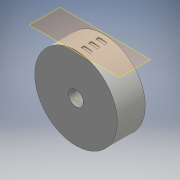
# Autodesk Inventor part: Part4
Saved by Autodesk Inventor 2016 (Build 200138000, 138)
## iProperties
Created: 2016-09-09
Part Number: Part4
Material: Generic
Document SubType Name: Modeling
Designer: Muhammad
Density: 1 g/cm^3
Appearance: Default
Author: Muhammad
Autodesk Inventor part; units mm, degrees
ref_plane "YZ Plane" through (0, 0, 0) normal (1, 0, 0) x (0, 1, 0)
ref_plane "XZ Plane" through (0, 0, 0) normal (0, 1, 0) x (-1, 0, 0)
sketch "Sketch1" plane through (0, 0, 0) normal (0, 1, 0) x (-1, 0, 0)
  circle A0 centre (0, 0) radius 14
  circle A1 centre (0, 0) radius 2.5
  dimension "d0" = 28
  dimension "d1" = 5
  constraints: 2 centre point, 2 coincident
  measures "d0" diameter of A0
  measures "d1" diameter of A1
extrude "Extrusion1" add sketch "Sketch1" along normal blind 9.5
sketch "Sketch2" plane through (0, 0, 0) normal (0, 0, 1) x (1, 0, 0)
  point P0 (0, 0)
ref_plane "Work Plane1" through (0, 0, 14) normal (0, 0, 1) x (1, 0, 0)
sketch "Sketch3" plane through (0, 0, 14) normal (0, 0, 1) x (1, 0, 0)
  line L0 (14, 9.5) -> (-14, 9.5) construction
  line L1 (0, 4.75) -> (14.9722, 4.75) construction
  line L2 (14.9722, 4.75) -> (-13.3278, 4.75) construction
  line L3 (0, 4.75) -> (0, 5.25) construction
  line L4 (0, 5.25) -> (4.1506, 5.25)
  line L5 (0, 4.75) -> (0, 4.25) construction
  line L6 (0, 4.25) -> (4.1506, 4.25) construction
  line L7 (4.1506, 4.25) -> (4.1506, 5.25) construction
  line L8 (0, 5.25) -> (0, 4.25) construction
  line L9 (0, 4.75) -> (0, 7.25) construction
  line L10 (0, 4.75) -> (0, 2.25) construction
  line L11 (0, 7.25) -> (0, 7.75) construction
  line L12 (0, 7.75) -> (4.1506, 7.75)
  line L13 (4.1506, 7.75) -> (4.1506, 6.75)
  line L14 (4.1506, 6.75) -> (0, 6.75)
  line L15 (0, 6.75) -> (0, 7.75)
  line L16 (0, 1.75) -> (4.1506, 1.75)
  line L17 (4.1506, 1.75) -> (4.1506, 2.75)
  line L18 (4.1506, 2.75) -> (0, 2.75)
  line L19 (0, 2.75) -> (0, 1.75)
  line L20 (4.1506, 5.25) -> (4.1506, 4.25)
  line L21 (0, 4.25) -> (4.1506, 4.25)
  line L22 (0, 5.25) -> (0, 4.25)
  point P0 (0, 0)
  dimension "d12" = 0.5
  dimension "d13" = 1
  constraints: 44 end point, 4 collinear, 4 symmetric about line, 3 horizontal, 3 perpendicular, 3 vertical, 2 parallel, 2 point on line
  measures "d12" distance of L9.end L11.end
  measures "d13" distance of L12.end L13.end
extrude "Extrusion2" cut sketch "Sketch3" against normal blind 0.3
body "Solid1"
